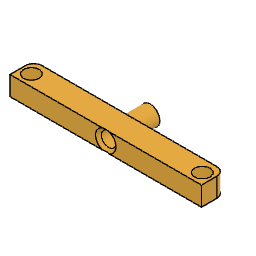
Com Magnet holder (Autodesk Fusion 360 design; units mm, degrees)
Autodesk Fusion 360 part; units mm, degrees
sketch "Commutator_Bottom_V1" plane through (0, 0, 0) normal (0, 1, 0) x (1, 0, 0)
sketch "Sketch2" plane through (0, 0, 0) normal (0, 1, 0) x (1, 0, 0)
  circle A0 centre (-3, -2) radius 29
  line L0 (11.8545, 12.9999) -> (-17.9527, 12.9999)
  line L1 (-3, -2) -> (13.5302, 15.2562)
  line L2 (-3, -2) -> (-20.1121, 14.3922)
  line L3 (-20.1121, 14.3922) -> (-20.1121, -3.2941)
  line L4 (-20.1121, -3.2941) -> (-3, -2)
  line L5 (13.5302, 15.2562) -> (13.5302, -4.0945)
  line L6 (13.5302, -4.0945) -> (-3, -2)
  line L7 (-128.5, 3) -> (-82.5, 3)
  line L8 (-82.5, 3) -> (-82.5, -3)
  line L9 (-82.5, -3) -> (-128.5, -3)
  line L10 (-128.5, -3) -> (-128.5, 3)
  line L11 (-128.5, 3) -> (-82.5, -3) construction
  line L12 (-82.5, 3) -> (-128.5, -3) construction
  line L13 (-17.9527, 12.9999) -> (-17.778, -3.1176)
  line L14 (11.8545, 12.9999) -> (11.2998, -3.8119)
  line L15 (-105.5, 0) -> (-126.06, 0)
  line L16 (-105.5, 0) -> (-85, 0)
  circle A1 centre (-126.06, 0) radius 1.65
  circle A2 centre (-85, 0) radius 1.65
  line L17 (11.17, -12.9044) -> (-14.3912, 11.7817)
  line L18 (-14.3912, 11.7817) -> (-17.17, 8.9044)
  line L19 (-17.17, 8.9044) -> (8.3912, -15.7817)
  line L20 (8.3912, -15.7817) -> (11.17, -12.9044)
  line L21 (11.17, -12.9044) -> (-17.17, 8.9044) construction
  line L22 (-14.3912, 11.7817) -> (8.3912, -15.7817) construction
  line L23 (11.7989, 11.3143) -> (-17.9309, 10.9921)
  line L24 (11.7989, 11.3143) -> (12.6076, 11.3231)
  line L25 (12.6076, 11.3231) -> (16.094, 11.3609)
  line L26 (16.094, 11.3609) -> (-20.891, 10.96)
  point P0 (-105.5, 0)
  point P1 (-3, -2)
  dimension "d1" = 58
  dimension "d2" = 46
  dimension "d3" = 6
  dimension "d4" = 20.56
  dimension "d5" = 20.5
  dimension "d6" = 3.3
  dimension "d7" = 3.3
  dimension "d23" = 4
  constraint horizontal L0
  constraint coincident A0.centre L1.start
  constraint perpendicular L1 L2
  constraint vertical L3
  constraint perpendicular L0 L5
  constraint horizontal L7
  constraint perpendicular L7 L8
  constraint parallel L7 L9
  constraint parallel L8 L10
  constraint coincident L11 P0
  constraint coincident L12 P0
  constraint coincident L4 L13.end
  constraint coincident L6 L14.end
  constraint coincident P0 L15.start
  constraint parallel L9 L15
  constraint parallel L15 L16
  constraint coincident L15.end A1.centre
  constraint coincident L16.end A2.centre
  constraint perpendicular L17 L18
  constraint parallel L17 L19
  constraint parallel L18 L20
  constraint coincident L21 P1
  constraint coincident L22 P1
  constraint coincident P1 A0.centre
  constraint coincident L14 L23.start
  constraint coincident L13 L23.end
  constraint perpendicular L13 L23
  measures "d1" diameter of A0
  measures "d2" distance of L8.end L9.end
  measures "d3" distance of L7.end L8.end
  measures "d4" distance of P0 L15.end
  measures "d5" distance of P0 L16.end
  measures "d6" diameter of A1
  measures "d7" diameter of A2
  measures "d23" distance of L17.end L18.end
extrude "Extrude1" add sketch "Sketch2" along normal blind 5 contours L7 L8 L9 L10
sketch "Sketch3" plane through (0, 0, -3) normal (0, 0, -1) x (-1, 0, 0)
  line L0 (82.5, 0) -> (128.5, 0)
  line L1 (128.5, 0) -> (128.5, 5)
  line L2 (128.5, 5) -> (82.5, 5)
  line L3 (82.5, 5) -> (82.5, 0)
  circle A0 centre (105.5, 2.5) radius 2.5
  circle A1 centre (105.5, 2.5) radius 1.75
  line L4 (82.5, 2.5) -> (105.5, 2.5)
  dimension "d10" = 5
  dimension "d11" = 3.5
  dimension "d24" = 23
  constraint concentric A0 A1
  constraint midpoint L3 L4.start
  constraint perpendicular L3 L4
  constraint coincident A0.centre A1.centre
  measures "d10" diameter of A0
  measures "d11" diameter of A1
  measures "d24" distance of L4.start A0.centre
extrude "Extrude2" add sketch "Sketch3" along normal blind 5 contours A0
extrude "Extrude3" cut 1 faces at (-105.8637, 2.9561, -3) along direction (0, 0, 1) blind 15
fillet "Fillet1" radius 2 4 edges at (-128.5, 2.5, 3) (-128.5, 2.5, -3) (-82.5, 2.5, 3) (-82.5, 2.5, -3)
hole "Hole1" at (-105.5, 2.5, 3) direction (0, 0, -1) diameter 3.5 depth 34.375 tip angle 118 countersink diameter 5.5 countersink angle 90
delete_face "DeleteFace1" 1 faces at (-82.8708, 1.6667, 2.1601)
delete_face "DeleteFace2" 1 faces at (-126.8785, 1.6667, 2.9639)
move_face "OffsetFaces1" offset -0.2 2 faces at (-126.8127, 3.3333, -1.4683) (-85.6786, 1.6667, -1.504)
extrude "Extrude4" cut 2 faces at (-121.75, 2.5, 3) (-89.25, 2.5, 3) along direction (0, 0, -1) blind 0.3
delete_face "DeleteFace3" 1 faces at (-106.7632, 0.0573, 2.9)
extrude "Extrude5" cut 1 faces at (-103.7186, 1.1352, -8) along direction (0, 0, 1) blind 1
extrude "Extrude6" add 1 faces at (-103.7186, 1.1352, -7) along direction (0, 0, -1) blind 1
move_face "OffsetFaces2" offset -0.2 1 faces at (-104.0917, 4.5656, -6.3333)
extrude "Extrude7" cut 1 faces at (-99.0512, 0, -2.4821) along direction (0, 1, 0) blind 0.2
move_face "OffsetFaces3" offset -0.2 1 faces at (-99.0512, 5, -2.4821)
equation "d2 = ( 23 * 2 ) * 1 mm"
named bodies: "Com_MagnetMount"
